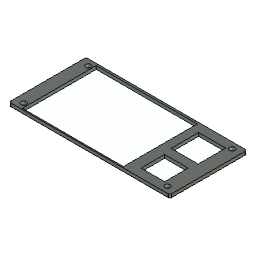
front_plate (Autodesk Fusion 360 design; units mm, degrees)
part number: 2025-12-15-21-06-19-821
Autodesk Fusion 360 part; units mm, degrees
sketch "Sketch1" plane through (0, 0, 0) normal (0, 0, 1) x (1, 0, 0)
  line L0 (0, 0) -> (96, 0)
  line L1 (96, 0) -> (96, 46)
  line L2 (96, 46) -> (0, 46)
  line L3 (0, 46) -> (0, 0)
  dimension "d1" = 96
  dimension "d2" = 46
  constraint horizontal L0
  constraint vertical L1
  constraint horizontal L2
  constraint vertical L3
  measures "d1" distance of L0.start L0.end
  measures "d2" distance of L0.start L2.end
extrude "Extrude1" add sketch "Sketch1" along normal blind 2
fillet "Fillet1" radius 1 4 edges at (96, 0, 1) (96, 46, 1) (0, 46, 1) (0, 0, 1)
sketch "Sketch2" plane through (0, 0, 2) normal (0, 0, 1) x (-1, 0, 0)
  arc A0 (0, -1) -> (-1, 0) centre (-1, -1) ccw
  line L0 (-1, 0) -> (-95, 0)
  arc A1 (-95, 0) -> (-96, -1) centre (-95, -1) ccw
  line L1 (-96, -1) -> (-96, -45)
  arc A2 (-96, -45) -> (-95, -46) centre (-95, -45) ccw
  line L2 (-95, -46) -> (-1, -46)
  arc A3 (-1, -46) -> (0, -45) centre (-1, -45) ccw
  line L3 (0, -45) -> (0, -1)
  circle A4 centre (-5.1, -42.25) radius 1.6
  circle A5 centre (-90.9, -42.25) radius 1.6
  circle A6 centre (-90.9, -3.75) radius 1.6
  circle A7 centre (-5.1, -3.75) radius 1.6
  dimension "d7" = 3.2
  dimension "d8" = 3.75
  dimension "d9" = 5.1
  dimension "d10" = 3.2
  dimension "d11" = 3.2
  dimension "d12" = 3.2
  dimension "d13" = 3.75
  dimension "d14" = 5.1
  dimension "d15" = 3.75
  dimension "d16" = 5.1
  dimension "d17" = 5.1
  dimension "d18" = 3.75
  measures "d7" diameter of A4
  measures "d8" distance of L2 A4.centre
  measures "d9" distance of L3 A4.centre
  measures "d10" diameter of A5
  measures "d11" diameter of A6
  measures "d12" diameter of A7
  measures "d13" distance of L0 A7.centre
  measures "d14" distance of L3 A7.centre
  measures "d15" distance of L0 A6.centre
  measures "d16" distance of L1 A6.centre
  measures "d17" distance of L1 A5.centre
  measures "d18" distance of L2 A5.centre
extrude "Extrude2" cut sketch "Sketch2" against normal blind 2 contours A4 | A5 | A6 | A7
sketch "Sketch3" plane through (0, 0, 2) normal (0, 0, 1) x (-1, 0, 0)
  circle A0 centre (-90.9, -3.75) radius 1.6
  circle A1 centre (-5.1, -3.75) radius 1.6
  circle A2 centre (-90.9, -42.25) radius 1.6
  circle A3 centre (-5.1, -42.25) radius 1.6
  arc A4 (0, -1) -> (-1, 0) centre (-1, -1) ccw
  line L0 (-1, 0) -> (-95, 0)
  arc A5 (-95, 0) -> (-96, -1) centre (-95, -1) ccw
  line L1 (-96, -1) -> (-96, -45)
  arc A6 (-96, -45) -> (-95, -46) centre (-95, -45) ccw
  line L2 (-95, -46) -> (-1, -46)
  arc A7 (-1, -46) -> (0, -45) centre (-1, -45) ccw
  line L3 (0, -45) -> (0, -1)
  line L4 (-2.5, -46) -> (-2.5, 0) construction
  line L5 (-7.3, -46) -> (-7.3, 0)
  line L6 (-93.5, -46) -> (-93.5, 0)
  line L7 (-88.5, -46) -> (-88.5, 0)
  line L8 (-7.3, -44.75) -> (-67.5, -44.75)
  line L9 (-67.5, -44.75) -> (-67.5, -0.75)
  line L10 (-67.5, -0.75) -> (-7.3, -0.75)
  line L11 (-7.3, -0.75) -> (-7.3, -44.75)
  line L12 (0, -23) -> (-96, -23) construction
  dimension "d21" = 2.6
  dimension "d22" = 4.8
  dimension "d23" = 2.6
  dimension "d24" = 5
  dimension "d26" = 44
  dimension "d27" = 44
  dimension "d29" = 21.75
  dimension "d30" = 22
  dimension "d31" = 4.8
  dimension "d32" = 21
  dimension "d34" = 60.2
  constraint coincident L2 L4.start
  constraint perpendicular L2 L4
  constraint coincident L0 L4.end
  constraint coincident L2 L5.start
  constraint perpendicular L2 L5
  constraint coincident L0 L5.end
  constraint coincident L2 L6.start
  constraint coincident L0 L6.end
  constraint coincident L2 L7.start
  constraint coincident L0 L7.end
  constraint perpendicular L0 L7
  constraint horizontal L8
  constraint vertical L9
  constraint horizontal L10
  constraint vertical L11
  constraint coincident L3 L12.start
  constraint coincident L1 L12.end
  constraint perpendicular L1 L12
  measures "d21" distance of A3.centre L4
  measures "d22" distance of L4 L5
  measures "d23" distance of A0.centre L6
  measures "d24" distance of L6 L7
  measures "d26" distance of L8.start L10.end
  measures "d27" distance of A5.end L1.end
  measures "d29" distance of L8 L12
  measures "d30" distance of A7.end L12
  measures "d31" distance of L4 L11
  measures "d32" distance of L7 L9
  measures "d34" distance of L5 L9
extrude "Extrude3" cut sketch "Sketch3" against normal blind 2 contours L5 L8 L9 L10 L11
sketch "Sketch4" plane through (0, 0, 2) normal (0, 0, 1) x (-1, 0, 0)
  line L0 (-67.5, -44.75) -> (-67.5, -0.75)
  line L1 (-67.5, -0.75) -> (-7.3, -0.75)
  line L2 (-7.3, -0.75) -> (-7.3, -44.75)
  line L3 (-7.3, -44.75) -> (-67.5, -44.75)
  circle A0 centre (-90.9, -3.75) radius 1.6
  circle A1 centre (-5.1, -3.75) radius 1.6
  circle A2 centre (-90.9, -42.25) radius 1.6
  circle A3 centre (-5.1, -42.25) radius 1.6
  arc A4 (0, -1) -> (-1, 0) centre (-1, -1) ccw
  line L4 (-1, 0) -> (-95, 0)
  arc A5 (-95, 0) -> (-96, -1) centre (-95, -1) ccw
  line L5 (-96, -1) -> (-96, -45)
  arc A6 (-96, -45) -> (-95, -46) centre (-95, -45) ccw
  line L6 (-95, -46) -> (-1, -46)
  arc A7 (-1, -46) -> (0, -45) centre (-1, -45) ccw
  line L7 (0, -45) -> (0, -1)
  line L8 (-93.5, -46) -> (-93.5, 0)
  line L9 (-88.5, -46) -> (-88.5, 0)
  line L10 (-73.4, -39.75) -> (-87.8, -39.75)
  line L11 (-87.8, -39.75) -> (-87.8, -25.35)
  line L12 (-87.8, -25.35) -> (-73.4, -25.35)
  line L13 (-73.4, -25.35) -> (-73.4, -39.75)
  line L14 (-74.6, -18.25) -> (-86.6, -18.25)
  line L15 (-86.6, -18.25) -> (-86.6, -6.25)
  line L16 (-86.6, -6.25) -> (-74.6, -6.25)
  line L17 (-74.6, -6.25) -> (-74.6, -18.25)
  line L18 (-72.4, -40.75) -> (-88.8, -40.75)
  line L19 (-88.8, -40.75) -> (-88.8, -24.35)
  line L20 (-88.8, -24.35) -> (-72.4, -24.35)
  line L21 (-72.4, -24.35) -> (-72.4, -40.75)
  line L22 (-73.6, -5.25) -> (-73.6, -19.25)
  line L23 (-73.6, -19.25) -> (-87.6, -19.25)
  line L24 (-87.6, -19.25) -> (-87.6, -5.25)
  line L25 (-87.6, -5.25) -> (-73.6, -5.25)
  dimension "d38" = 2.6
  dimension "d39" = 5
  dimension "d40" = 14.4
  dimension "d41" = 14.4
  dimension "d42" = 5.7
  dimension "d44" = 12
  dimension "d45" = 12
  dimension "d46" = 6.9
  dimension "d47" = 7.1
  dimension "d48" = -1
  dimension "d49" = -1
  dimension "d50" = 5
  constraint coincident L6 L8.start
  constraint coincident L4 L8.end
  constraint perpendicular L4 L8
  constraint coincident L6 L9.start
  constraint coincident L4 L9.end
  constraint perpendicular L4 L9
  constraint horizontal L10
  constraint vertical L11
  constraint horizontal L12
  constraint vertical L13
  constraint horizontal L14
  constraint vertical L15
  constraint horizontal L16
  constraint vertical L17
  measures "d38" distance of A2.centre L8
  measures "d39" distance of L8 L9
  measures "d40" distance of L10.start L10.end
  measures "d41" distance of L10.start L12.end
  measures "d42" distance of L8 L11
  measures "d44" distance of L14.start L14.end
  measures "d45" distance of L14.start L16.end
  measures "d46" distance of L8 L15
  measures "d47" distance of L12 L14
  measures "d50" distance of L3 L10
extrude "Extrude4" cut sketch "Sketch4" against normal blind 2 contours L9 L18 L20 L21 | L10 L11 L12 L13 | L14 L15 L16 L17 | L22 L23 L24 L25
sketch "Sketch5" plane through (0, 0, 2) normal (0, 0, 1) x (-1, 0, 0)
  line L0 (-88.5, -40.75) -> (-88.5, -24.35)
  line L1 (-88.5, -24.35) -> (-72.4, -24.35)
  line L2 (-72.4, -24.35) -> (-72.4, -40.75)
  line L3 (-72.4, -40.75) -> (-88.5, -40.75)
  line L4 (-73.6, -19.25) -> (-87.6, -19.25)
  line L5 (-87.6, -19.25) -> (-87.6, -5.25)
  line L6 (-87.6, -5.25) -> (-73.6, -5.25)
  line L7 (-73.6, -5.25) -> (-73.6, -19.25)
  line L8 (-67.5, -44.75) -> (-67.5, -0.75)
  line L9 (-67.5, -0.75) -> (-7.3, -0.75)
  line L10 (-7.3, -0.75) -> (-7.3, -44.75)
  line L11 (-7.3, -44.75) -> (-67.5, -44.75)
  circle A0 centre (-90.9, -3.75) radius 1.6
  circle A1 centre (-5.1, -3.75) radius 1.6
  circle A2 centre (-90.9, -42.25) radius 1.6
  circle A3 centre (-5.1, -42.25) radius 1.6
  arc A4 (0, -1) -> (-1, 0) centre (-1, -1) ccw
  line L12 (-1, 0) -> (-95, 0)
  arc A5 (-95, 0) -> (-96, -1) centre (-95, -1) ccw
  line L13 (-96, -1) -> (-96, -45)
  arc A6 (-96, -45) -> (-95, -46) centre (-95, -45) ccw
  line L14 (-95, -46) -> (-1, -46)
  arc A7 (-1, -46) -> (0, -45) centre (-1, -45) ccw
  line L15 (0, -45) -> (0, -1)
  dimension "d53" = 3.75
  dimension "d54" = 3.75
  dimension "d55" = 3.75
  measures "d53" distance of A1.centre L12
  measures "d54" distance of A2.centre L14
  measures "d55" distance of A0.centre L12
equation "d21 = 1 mm + ( ( 3.2 / 2 ) * 1 mm )"
equation "d29 = ( 43.5 / 2 ) * 1 mm"
equation "d38 = ( 3.2 / 2 ) * 1 mm + 1 mm"
